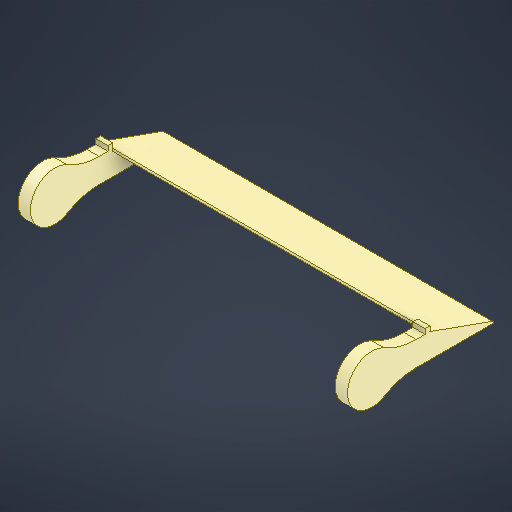
# Autodesk Inventor part: cuchilla
Saved by Autodesk Inventor 2026.2 (Build 302298010, 298A)
## iProperties
Created: 2026-05-09
Part Number: cuchilla
Material: Genérico
Document SubType Name: Modeling
Designer: migue
Density: 1 g/cm^3
Appearance: Nilón 6
Author: migue
Autodesk Inventor part; units mm, degrees
ref_plane "YZ Plane" through (0, 0, 0) normal (1, 0, 0) x (0, 1, 0)
ref_plane "XZ Plane" through (0, 0, 0) normal (0, 1, 0) x (-1, 0, 0)
sketch "Boceto1" plane through (0, 0, 0) normal (1, 0, 0) x (0, 1, 0)
  arc A0 (8.5318, -5.2161) -> (-8.461, -5.3303) centre (0, 0) ccw
  line L0 (-5, -17.956) -> (-5, -50)
  line L1 (-5, -50) -> (-4.3301, -50)
  line L2 (5, -21.8397) -> (5, -18.1978)
  line L3 (0, 0) -> (8.6603, -5) construction
  line L4 (0, 0) -> (10, 0) construction
  line L5 (0, 0) -> (-8.6603, -5) construction
  line L6 (0, 0) -> (10, 0) construction
  arc A1 (8.6603, -5) -> (5, -18.1978) centre (30.624, -18.1978) ccw
  arc A2 (-5, -17.956) -> (-8.6603, -5) centre (-29.7601, -17.956) ccw
  line L7 (-4.3301, -50) -> (5, -23.8397)
  line L8 (5, -23.8397) -> (7, -23.8397)
  line L9 (7, -23.8397) -> (7, -21.8397)
  line L10 (7, -21.8397) -> (5, -21.8397)
  point P0 (-4.6651, -50)
  dimension "d3" = 30
  dimension "d4" = 210
  dimension "d8" = 50
  dimension "d16" = 10
  constraints: 22 end point, 10 point on circle, 3 centre point, 3 horizontal, 2 equal length, 2 parallel, 2 tangent, 1 coincident, 1 midpoint, 1 perpendicular
  measures "d3" angle of L3 L4
  measures "d8" vertical distance of point (-4.665, -50) point (0, 0)
  measures "d16" radius of A0
extrude "Extrusión1" add sketch "Boceto1" along normal blind 5
sketch "Boceto3" plane through (5, 0, 0) normal (1, 0, 0) x (0, 0, -1)
  line L0 (23.8397, 5) -> (50, -4.3301)
  line L1 (23.8397, 3.9383) -> (48.9014, -5)
  line L2 (17.956, -5) -> (50, -5) projected
  line L3 (50, -4.3301) -> (50, -5)
  line L4 (48.9014, -5) -> (50, -5)
  line L5 (23.8397, 3.9383) -> (23.8397, 5)
  point P0 (0, 0)
  dimension "d12" = 1
  constraints: 10 end point, 1 collinear, 1 horizontal alignment, 1 parallel, 1 perpendicular, 1 vertical, 1 vertical alignment
  measures "d12" distance between parallel lines of L0 L1
extrude "Extrusión2" add sketch "Boceto3" along normal blind 125
ref_plane "Plano de trabajo1" through (67.5, 0, 0) normal (1, 0, 0) x (0, 0, -1)
mirror "Simetría1" about plane through (67.5, 0, 0) normal (1, 0, 0) of "Extrusión1"
fillet "Empalme1" radius 1 1 edges at (67.5, -4.3301, -50)
